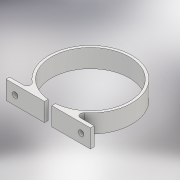
# Autodesk Inventor part: OmegaRing
Saved by Autodesk Inventor 2018 (Build 220112000, 112)
## iProperties
Created: 2018-03-27
Part Number: OmegaRing
Material: ABS Plastic
Document SubType Name: Modeling
Designer: mansu
Density: 1.06 g/cm^3
Appearance: Smooth - White
Author: mansu
Autodesk Inventor part; units mm, degrees
ref_plane "YZ Plane" through (0, 0, 0) normal (1, 0, 0) x (0, 1, 0)
ref_plane "XZ Plane" through (0, 0, 0) normal (0, 1, 0) x (-1, 0, 0)
ref_plane "XY Plane" through (0, 0, 0) normal (0, 0, 1) x (1, 0, 0)
sketch "Sketch1" plane through (0, 0, 0) normal (0, 0, 1) x (1, 0, 0)
  circle A0 centre (0, 0) radius 21.15 construction
  line L0 (-18, -23) -> (18, -23) construction
  line L1 (-18, -23) -> (-18, -38.1522) construction
  line L2 (18, -23) -> (18, -38.1522) construction
  line L3 (-23, -21) -> (-23, -23)
  line L4 (-23, -23) -> (-2, -23)
  line L5 (-2, -21.0552) -> (-2, -23)
  line L6 (2, -21.0552) -> (2, -23)
  line L7 (2, -23) -> (23, -23)
  line L8 (23, -23) -> (23, -21)
  line L9 (23, -21) -> (15.5468, -21)
  line L10 (-23, -21) -> (-15.5468, -21)
  arc A1 (14.2802, -17.4521) -> (-14.2802, -17.4521) centre (0, 0) ccw
  arc A2 (2, -21.0552) -> (-2, -21.0552) centre (0, 0) ccw
  arc A3 (14.2802, -17.4521) -> (15.5468, -21) centre (15.5468, -19) ccw
  arc A4 (-15.5468, -21) -> (-14.2802, -17.4521) centre (-15.5468, -19) ccw
  point P0 (0, -23)
  point P1 (8.216, -21)
  point P2 (-8.216, -21)
  dimension "d13" = 42.3
  dimension "d1" = 23
  dimension "d2" = 36
  dimension "d3" = 2
  dimension "d4" = 1.4
  dimension "d5" = 5
  dimension "d6" = 2
  dimension "d7" = 4
  constraints: 22 end point, 10 point on circle, 6 point on line, 5 perpendicular, 4 centre point, 4 tangent, 2 horizontal, 2 horizontal alignment, 2 vertical, 1 coincident, 1 collinear, 1 concentric, 1 equal radius, 1 midpoint, 1 vertical alignment, 4 other
  measures "d1" distance from line of point (0, 0) L0
  measures "d2" distance of L0.start L0.end
  measures "d3" distance of L7.end L8.end
  measures "d5" distance between parallel lines of L1 L3
  measures "d6" radius of A3
  measures "d7" distance between parallel lines of L5 L6
extrude "Extrusion1" add sketch "Sketch1" along normal blind 10
sketch "Sketch2" plane through (2, -23, 0) normal (0, -1, 0) x (1, 0, 0)
  circle A0 centre (16, 5) radius 1.5
  line L0 (21, 0) -> (21, 10) projected
  point P0 (-2, 0)
  point P1 (16, 0)
  point P2 (16, 0)
  point P3 (16, 0)
  point P4 (21, 5)
  dimension "d10" = 3
  constraints: 1 centre point, 1 horizontal alignment, 1 midpoint, 1 vertical alignment
  measures "d10" diameter of A0
extrude "Extrusion2" cut sketch "Sketch2" against normal up to surface (2 mm away)
mirror "Mirror1" about plane through (0, 0, 0) normal (1, 0, 0) of "Extrusion2"
body "Solid1"
